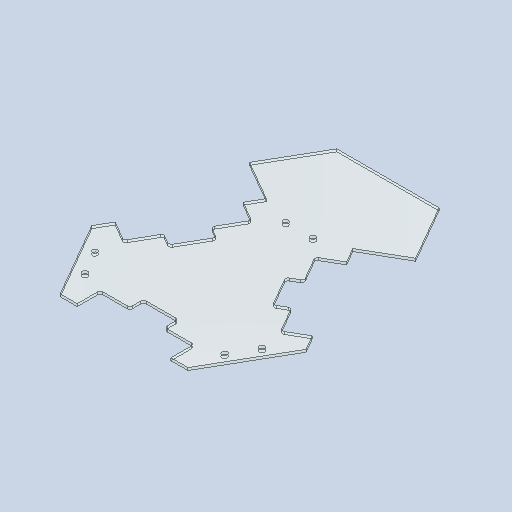
# Autodesk Inventor part: base_plate
Saved by Autodesk Inventor 2024.1 (Build 281209000, 209)
## iProperties
Created: 2025-02-03
Part Number: base_plate
Material: ガラス
Document SubType Name: Sheet Metal
Designer: hibik
Density: 2.18 g/cm^3
Sheet Metal Rule: Default_mm
Appearance: クリア
Author: hibik
Autodesk Inventor part; units mm, degrees
ref_plane "YZ Plane" through (0, 0, 0) normal (1, 0, 0) x (0, 1, 0)
ref_plane "XZ Plane" through (0, 0, 0) normal (0, 1, 0) x (-1, 0, 0)
ref_plane "XY Plane" through (0, 0, 0) normal (0, 0, 1) x (1, 0, 0)
sketch "スケッチ1" plane through (0, 0, 0) normal (0, 1, 0) x (-1, 0, 0)
  line L0 (75, 0) -> (105, -51.9615)
  line L1 (-75, 0) -> (-105, -51.9615)
  line L2 (0, -218.2384) -> (0, 36.3731)
  line L3 (147, 0) -> (-147, 0)
  line L4 (37.5, -27) -> (-37.5, -27)
  line L5 (105, -51.9615) -> (30, -181.8653)
  line L6 (30, -181.8653) -> (-30, -181.8653)
  line L7 (-30, -181.8653) -> (-105, -51.9615)
  line L8 (75, 0) -> (-75, 0)
  line L9 (-25.3673, -135.8894) -> (-62.8673, -70.9375)
  line L10 (25.3673, -135.8894) -> (62.8673, -70.9375)
  line L11 (-37.5, -27) -> (-27.5, -27)
  line L12 (-27.5, -27) -> (-27.5, -39)
  line L13 (-27.5, -39) -> (-37.5, -39)
  line L14 (-37.5, -39) -> (-37.5, -27)
  line L15 (37.5, -27) -> (27.5, -27)
  line L16 (27.5, -27) -> (27.5, -39)
  line L17 (27.5, -39) -> (37.5, -39)
  line L18 (37.5, -39) -> (37.5, -27)
  line L19 (0, -77.9423) -> (44.1173, -103.4134) construction
  line L20 (0, -77.9423) -> (-44.1173, -103.4134) construction
  line L21 (-44.1173, -103.4134) -> (-67.5, -116.9134) construction
  line L22 (-57.8673, -79.5977) -> (-47.475, -73.5977)
  line L23 (-52.475, -64.9375) -> (-62.8673, -70.9375)
  line L24 (-62.8673, -70.9375) -> (-57.8673, -79.5977)
  line L25 (-47.475, -73.5977) -> (-52.475, -64.9375)
  line L26 (-25.3673, -135.8894) -> (-30.3673, -127.2291)
  line L27 (-19.975, -121.2291) -> (-14.975, -129.8894)
  line L28 (-14.975, -129.8894) -> (-25.3673, -135.8894)
  line L29 (-30.3673, -127.2291) -> (-19.975, -121.2291)
  line L30 (30.3673, -127.2291) -> (19.975, -121.2291)
  line L31 (14.975, -129.8894) -> (25.3673, -135.8894)
  line L32 (25.3673, -135.8894) -> (30.3673, -127.2291)
  line L33 (19.975, -121.2291) -> (14.975, -129.8894)
  line L34 (62.8673, -70.9375) -> (57.8673, -79.5977)
  line L35 (47.475, -73.5977) -> (52.475, -64.9375)
  line L36 (52.475, -64.9375) -> (62.8673, -70.9375)
  line L37 (57.8673, -79.5977) -> (47.475, -73.5977)
  line L38 (62.8673, -70.9375) -> (37.5, -27)
  line L39 (-37.5, -27) -> (-62.8673, -70.9375)
  line L40 (-25.3673, -135.8894) -> (25.3673, -135.8894)
  line L41 (-25.3673, -135.8894) -> (-25.3673, -181.8653)
  line L42 (25.3673, -135.8894) -> (25.3673, -181.8653)
  line L43 (-25.3673, -135.8894) -> (-48.75, -149.3894)
  line L44 (25.3673, -135.8894) -> (48.75, -149.3894)
  point P0 (0, 0)
  point P1 (0, 0)
  point P2 (0, -27)
  dimension "d1" = 150
  dimension "d2" = 60
  dimension "d3" = 60
  dimension "d4" = 27
  dimension "d5" = 75
  dimension "d6" = 60
  dimension "d7" = 27
  dimension "d8" = 10
  dimension "d9" = 12
  dimension "d10" = 10
  dimension "d11" = 12
  dimension "d14" = 360
  measures "d1" distance of L1.start L0.start
  measures "d2" angle of L3 L0
  measures "d3" angle of L1 L3
  measures "d4" distance between parallel lines of L3 L4
  measures "d5" distance of L4.start L4.end
  measures "d6" distance of L5.end L6.end
  measures "d7" distance between parallel lines of L7 L9
  measures "d8" distance of L12.end L13.end
  measures "d9" distance of L11.end L12.end
  measures "d10" distance of L17.end L16.end
  measures "d11" distance of L16.end L15.end
extrude "プレート1" add sketch "スケッチ1" along normal blind 1.5 contours L5 L6 L42 L44 | L4 L16 L17 L18 L38 L36 L35 L37 L10 L30 L33 L31 L40 L2 | L2 L40 L28 L27 L29 L9 L22 L25 L23 L39 L14 L13 L12 L4 | L31 L33 L30 L10 | L42 L6 L2 L40 | L2 L6 L41 L40 | L4 L18 L17 L16 | L12 L13 L14 L4 | L9 L29 L27 L28 | L41 L6 L7 L43 | L37 L35 L36 L10 | L23 L25 L22 L9
sketch "スケッチ2" plane through (0, 0, 0) normal (0, -1, 0) x (1, 0, 0)
  line L0 (23.3798, -38.55) -> (-23.3798, -38.55) projected
  line L1 (8.2, -46.6) -> (-8.2, -46.6) projected
  arc A0 (-21.1, -27) -> (-23.3798, -38.55) centre (-21.1, -33) ccw projected
  line L2 (-27.5, -27) -> (-27.5, -39) projected
  line L3 (27.5, -39) -> (27.5, -27) projected
  line L4 (-27.5, -39) -> (-27.5, -40.55)
  line L5 (-27.5, -40.55) -> (-10.2, -40.55)
  line L6 (-10.2, -40.55) -> (-10.2, -48.6)
  line L7 (-10.2, -48.6) -> (10.2, -48.6)
  line L8 (10.2, -48.6) -> (10.2, -40.55)
  line L9 (10.2, -40.55) -> (27.5, -40.55)
  line L10 (27.5, -40.55) -> (27.5, -39)
  line L11 (-37.5, -27) -> (-27.5, -27) projected
  line L12 (-37.5, -27) -> (37.5, -27) projected
  line L13 (-20.3112, -101.4469) -> (-30.5112, -83.78)
  line L14 (-27.2827, -105.4719) -> (-20.3112, -101.4469)
  line L15 (-18.6327, -120.4541) -> (-27.2827, -105.4719)
  line L16 (-19.975, -121.2291) -> (-18.6327, -120.4541)
  line L17 (-37.4827, -87.805) -> (-46.1327, -72.8227)
  line L18 (-46.1327, -72.8227) -> (-47.475, -73.5977)
  line L19 (-30.5112, -83.78) -> (-37.4827, -87.805)
  line L20 (30.5112, -83.78) -> (20.3112, -101.4469)
  line L21 (37.4827, -87.805) -> (30.5112, -83.78)
  line L22 (46.1327, -72.8227) -> (37.4827, -87.805)
  line L23 (47.475, -73.5977) -> (46.1327, -72.8227)
  line L24 (27.2827, -105.4719) -> (18.6327, -120.4541)
  line L25 (18.6327, -120.4541) -> (19.975, -121.2291)
  line L26 (20.3112, -101.4469) -> (27.2827, -105.4719)
  line L27 (-47.475, -73.5977) -> (-57.8673, -79.5977)
  line L28 (-57.8673, -79.5977) -> (-30.3673, -127.2291)
  line L29 (-30.3673, -127.2291) -> (-19.975, -121.2291)
  line L30 (19.975, -121.2291) -> (30.3673, -127.2291)
  line L31 (30.3673, -127.2291) -> (57.8673, -79.5977)
  line L32 (57.8673, -79.5977) -> (47.475, -73.5977)
  point P0 (0, 0)
  point P1 (0, -77.9423)
  point P2 (-23.0432, -100.7148)
  point P3 (-33.5673, -121.6866)
  point P4 (-22.4248, -117.8859)
  point P5 (-25.3673, -135.8894)
  point P6 (-28.3712, -118.6866)
  point P7 (-31.2432, -86.512)
  point P8 (-45.8046, -77.3909)
  point P9 (-62.8673, -70.9375)
  point P10 (31.2432, -86.512)
  point P11 (54.6673, -85.1403)
  point P12 (45.8046, -77.3909)
  point P13 (62.8673, -70.9375)
  point P14 (49.4712, -82.1403)
  point P15 (23.0432, -100.7148)
  point P16 (22.4248, -117.8859)
  point P17 (25.3673, -135.8894)
  dimension "d17" = 2
  dimension "d18" = 2
  dimension "d19" = 2
  dimension "d20" = 2
  dimension "d26" = 360
  constraints: 54 end point, 9 perpendicular, 1 collinear, 1 horizontal, 1 vertical, 76 other
  measures "d17" distance between parallel lines of L0 L5
  measures "d18" distance from line of L1.end L6
  measures "d19" distance from line of L8 L1.start
  measures "d20" distance between parallel lines of L7 L1
extrude "切り取り1" cut sketch "スケッチ2" against normal blind 1.5
fillet "フィレット1" radius 1.5 18 edges at (-10.2, 0.75, -48.6) (-10.2, 0.75, -40.55) (-27.5, 0.75, -40.55) (10.2, 0.75, -48.6) (10.2, 0.75, -40.55) (27.5, 0.75, -40.55) (-30.5112, 0.75, -83.78) (-46.1327, 0.75, -72.8227) (-20.3112, 0.75, -101.4469) (-27.2827, 0.75, -105.4719) (-37.4827, 0.75, -87.805) (-18.6327, 0.75, -120.4541) (20.3112, 0.75, -101.4469) (27.2827, 0.75, -105.4719) (18.6327, 0.75, -120.4541) (30.5112, 0.75, -83.78) (37.4827, 0.75, -87.805) (46.1327, 0.75, -72.8227)
sketch "スケッチ3" plane through (0, 0, 0) normal (0, -1, 0) x (1, 0, 0)
  circle A0 centre (40.9875, -45.0405) radius 1.6 projected
  circle A1 centre (48.9875, -58.8969) radius 1.6 projected
  circle A2 centre (8, -129.8894) radius 1.6 projected
  circle A3 centre (-8, -129.8894) radius 1.6 projected
  circle A4 centre (-48.9875, -58.8969) radius 1.6 projected
  circle A5 centre (-40.9875, -45.0405) radius 1.6 projected
  point P0 (0, 0)
extrude "切り取り2" cut sketch "スケッチ3" against normal blind 1.5
equation "\"d3\" = d2"
equation "\"d7\" = d4"
equation "\"d19\" = d18"
equation "\"d21\" = Thickness"
equation "\"d28\" = Thickness"
equation "\"d16\" = Thickness"
equation "\"BendRadius\" = Thickness"
equation "\"BendReliefWidth\" = Thickness"
equation "\"BendReliefDepth\" = 0.5 * Thickness"
equation "\"CornerReliefSize\" = 4 * Thickness"
equation "\"MinimumRemnant\" = 2 * Thickness"
equation "\"TransitionRadius\" = BendRadius"
equation "\"JacobiRadiusSize\" = BendRadius"
equation "\"GapSize\" = Thickness"
equation "\"Thickness\" = 1.5"
